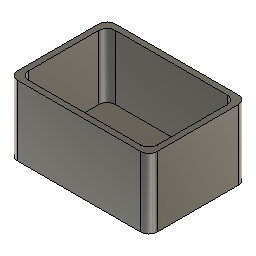
switch box v0 (Autodesk Fusion 360 design; units mm, degrees)
Autodesk Fusion 360 part; units mm, degrees
sketch "Sketch1" plane through (0, 0, 0) normal (0, 0, 1) x (1, 0, 0)
  line L0 (37.9069, 19.6511) -> (-12.0931, 19.6511)
  line L1 (-12.0931, 19.6511) -> (-12.0931, -15.3489)
  line L2 (-12.0931, -15.3489) -> (37.9069, -15.3489)
  line L3 (37.9069, -15.3489) -> (37.9069, 19.6511)
  dimension "d1" = 50
  dimension "d2" = 35
  constraint horizontal L0
  constraint vertical L1
  constraint horizontal L2
  constraint vertical L3
  measures "d1" distance of L0.start L0.end
  measures "d2" distance of L0.start L2.end
extrude "Extrude1" add sketch "Sketch1" along normal blind 25
shell "Shell1" thickness 2 removed faces 1 at (4.5736, 7.9845, 25)
fillet "Fillet1" radius 3 8 edges at (37.9069, -15.3489, 12.5) (37.9069, 19.6511, 12.5) (-10.0931, -13.3489, 13.5) (-12.0931, 19.6511, 12.5) (35.9069, 17.6511, 13.5) (-12.0931, -15.3489, 12.5) (-10.0931, 17.6511, 13.5) (35.9069, -13.3489, 13.5)
sketch "Sketch2" plane through (0, 0, 25) normal (0, 0, 1) x (-1, 0, 0)
  line L0 (-32.9069, 13.3489) -> (7.0931, 13.3489)
  arc A0 (10.0931, 10.3489) -> (7.0931, 13.3489) centre (7.0931, 10.3489) ccw
  line L1 (10.0931, 10.3489) -> (10.0931, -14.6511)
  arc A1 (7.0931, -17.6511) -> (10.0931, -14.6511) centre (7.0931, -14.6511) ccw
  line L2 (7.0931, -17.6511) -> (-32.9069, -17.6511)
  arc A2 (-35.9069, -14.6511) -> (-32.9069, -17.6511) centre (-32.9069, -14.6511) ccw
  line L3 (-35.9069, -14.6511) -> (-35.9069, 10.3489)
  arc A3 (-32.9069, 13.3489) -> (-35.9069, 10.3489) centre (-32.9069, 10.3489) ccw
  arc A4 (12.0931, 12.3489) -> (9.0931, 15.3489) centre (9.0931, 12.3489) ccw
  line L4 (9.0931, 15.3489) -> (-34.9069, 15.3489)
  arc A5 (-34.9069, 15.3489) -> (-37.9069, 12.3489) centre (-34.9069, 12.3489) ccw
  line L5 (-37.9069, 12.3489) -> (-37.9069, -16.6511)
  arc A6 (-37.9069, -16.6511) -> (-34.9069, -19.6511) centre (-34.9069, -16.6511) ccw
  line L6 (-34.9069, -19.6511) -> (9.0931, -19.6511)
  arc A7 (9.0931, -19.6511) -> (12.0931, -16.6511) centre (9.0931, -16.6511) ccw
  line L7 (12.0931, -16.6511) -> (12.0931, 12.3489)
  circle A8 centre (-21.6814, -1.7334) radius 3.5
  circle A9 centre (-3.3782, -1.7334) radius 3.5
  dimension "d8" = 7
  dimension "d9" = 7
  measures "d8" diameter of A8
  measures "d9" diameter of A9
extrude "Extrude2" cut sketch "Sketch2" against normal blind 60 contours A8 | A9
